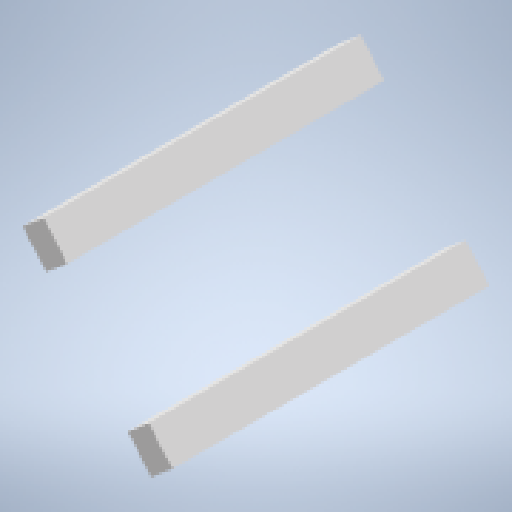
# Autodesk Inventor part: servo_holder
Saved by Autodesk Inventor 2024 (Build 280153000, 153)
## iProperties
Created: 2026-02-15
Part Number: servo_holder
Material: Generic
Document SubType Name: Modeling
Designer: SEMEN
Density: 1 g/cm^3
Appearance: Default
Author: SEMEN
Autodesk Inventor part; units mm, degrees
ref_plane "YZ Plane" through (0, 0, 0) normal (1, 0, 0) x (0, 1, 0)
ref_plane "XZ Plane" through (0, 0, 0) normal (0, 1, 0) x (-1, 0, 0)
ref_plane "XY Plane" through (0, 0, 0) normal (0, 0, 1) x (1, 0, 0)
sketch "Sketch1" plane through (0, 0, 0) normal (0, 0, 1) x (1, 0, 0)
  line L0 (90.2976, 72.8734) -> (70.813, 96.0776) projected
  line L1 (73.1601, 93.2824) -> (80.9715, 99.8416) projected
  line L2 (95.7618, 82.2278) -> (87.9505, 75.6686) projected
  line L3 (70.813, 96.0776) -> (68.8838, 98.3751)
  line L4 (68.8838, 98.3751) -> (74.2445, 102.8765)
  line L5 (74.2445, 102.8765) -> (78.5209, 97.7838)
  line L6 (90.2976, 72.8734) -> (92.2268, 70.5759)
  line L7 (92.2268, 70.5759) -> (97.5875, 75.0773)
  line L8 (97.5875, 75.0773) -> (93.3112, 80.17)
  line L9 (80.5553, 84.4755) -> (94.8669, 96.493) construction
  line L10 (90.9407, 72.1076) -> (89.2176, 70.6607) projected
  line L11 (94.9072, 72.8266) -> (90.6308, 77.9193) construction
  line L12 (71.5642, 100.6258) -> (75.8405, 95.5331) construction
  point P0 (0, 0)
  point P1 (92.769, 75.373)
  point P2 (73.7023, 98.0795)
  dimension "d0" = 2
  dimension "d1" = 7
  constraints: 18 end point, 7 point on line, 5 midpoint, 5 perpendicular, 1 other
  measures "d0" distance between parallel lines of L7 L10
  measures "d1" distance between parallel lines of L8 L0
ref_plane "Work Plane1" through (72.2806, 68.9104, 57.5461) normal (0, 0, 1) x (0.7658175, 0.643058, 0)
ref_plane "Work Plane2" through (75.6298, 74.8001, 12) normal (0, 0, 1) x (0.7658175, 0.643058, 0)
extrude "Extrusion1" add sketch "Sketch1" along normal up to surface (12 mm away)
sketch "Sketch2" plane through (97.5875, 75.0773, 12) normal (0, 0, 1) x (0.7658175, 0.643058, 0)
  line L0 (0, 0) -> (0, 6.65) projected
  line L1 (-7, 29.65) -> (-7, 36.3) projected
  line L2 (0, 0) -> (-7, 0)
  line L3 (-7, 0) -> (-7, 36.3)
  line L4 (-7, 36.3) -> (0, 36.3)
  line L5 (0, 36.3) -> (0, 0)
  point P0 (-123.0133, 5.2589)
  point P1 (0, 6.65)
  point P2 (-7, 29.65)
  constraints: 8 end point, 2 parallel, 1 horizontal, 1 perpendicular
extrude "Extrusion2" add sketch "Sketch2" along normal blind 4
hole "Hole1" at (73.7023, 98.0795, 0) at (92.769, 75.373, 0) direction (0, 0, 1) diameter 3.4 end through all clearance for "Countersunk Head GOST 12876-67" size "M3" standard "GOST"
fillet "Fillet1" radius 2 4 edges at (92.2268, 70.5759, 8) (97.5875, 75.0773, 8) (74.2445, 102.8765, 8) (68.8838, 98.3751, 8)
sketch "Sketch3" plane through (97.5875, 75.0773, 16) normal (0, 0, 1) x (0.7658175, 0.643058, 0)
  circle A0 centre (-3.5, 3.325) radius 1.7 projected
  circle A1 centre (-3.5, 32.975) radius 1.7 projected
  line L0 (-1.9123, 6.075) -> (-0.3246, 3.325)
  line L1 (-0.3246, 3.325) -> (-1.9123, 0.575)
  line L2 (-1.9123, 0.575) -> (-5.0877, 0.575)
  line L3 (-5.0877, 0.575) -> (-6.6754, 3.325)
  line L4 (-6.6754, 3.325) -> (-5.0877, 6.075)
  line L5 (-5.0877, 6.075) -> (-1.9123, 6.075)
  line L6 (-1.9123, 30.225) -> (-5.0877, 30.225)
  line L7 (-5.0877, 30.225) -> (-6.6754, 32.975)
  line L8 (-6.6754, 32.975) -> (-5.0877, 35.725)
  line L9 (-5.0877, 35.725) -> (-1.9123, 35.725)
  line L10 (-1.9123, 35.725) -> (-0.3246, 32.975)
  line L11 (-0.3246, 32.975) -> (-1.9123, 30.225)
  line L12 (-5, 0) -> (-2, 0) projected
  point P0 (-123.0133, 5.2589)
  point P1 (-3.5, 3.325)
  point P2 (-3.5, 32.975)
  dimension "d14" = 5.5
  dimension "d15" = 5.5
  constraints: 24 end point, 2 coincident, 2 parallel, 26 other
  measures "d14" distance between parallel lines of L2 L5
  measures "d15" distance between parallel lines of L9 L6
extrude "Extrusion3" cut sketch "Sketch3" against normal blind 2
body "Solid1"
